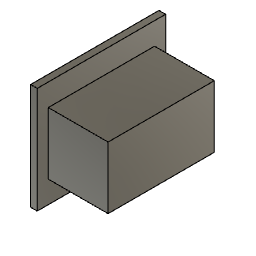
Assembly v11 (Autodesk Fusion 360 archive; units mm, degrees)
design "Power"
Autodesk Fusion 360 part; units mm, degrees
sketch "Sketch1" plane through (0, 0, 0) normal (1, 0, 0) x (0, 1, 0)
  line L0 (0, 0) -> (48, 0)
  line L1 (48, 0) -> (48, 28)
  line L2 (48, 28) -> (0, 28)
  line L3 (0, 28) -> (0, 0)
  dimension "d1" = 48
  dimension "d2" = 28
  constraint horizontal L0
  constraint vertical L1
  constraint horizontal L2
  constraint vertical L3
  constraint coincident L0.start L3.end
  measures "d1" distance of L0.start L0.end
  measures "d2" distance of L0.start L2.end
extrude "Extrude1" add sketch "Sketch1" along normal blind 27
sketch "Sketch2" plane through (0, 0, 0) normal (-1, 0, 0) x (0, -1, 0)
  line L0 (0, 0) -> (0, 28)
  line L1 (0, 28) -> (-48, 28)
  line L2 (-48, 28) -> (-48, 0)
  line L3 (-48, 0) -> (0, 0)
  line L4 (-48, 28) -> (0, 0) construction
  line L5 (0, 28) -> (-48, 0) construction
  line L6 (5, -10) -> (-53, -10)
  line L7 (-53, -10) -> (-53, 38)
  line L8 (-53, 38) -> (5, 38)
  line L9 (5, 38) -> (5, -10)
  line L10 (5, -10) -> (-53, 38) construction
  line L11 (-53, -10) -> (5, 38) construction
  point P0 (-24, 14)
  dimension "d5" = 58
  dimension "d6" = 48
  constraint coincident L1.end L2.start
  constraint coincident L0.start L3.end
  constraint coincident L0.end L1.start
  constraint coincident L2.end L3.start
  constraint horizontal L6
  constraint perpendicular L6 L7
  constraint parallel L6 L8
  constraint parallel L7 L9
  constraint coincident L10 P0
  constraint coincident L11 P0
  constraint midpoint L5 P0
  measures "d5" distance of L7.end L8.end
  measures "d6" distance of L6.end L7.end
extrude "Extrude2" add sketch "Sketch2" along normal blind 3 contours L0 L1 L2 L3 | L6 L7 L8 L9

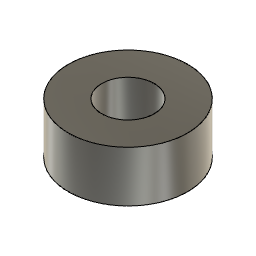
design "Transfo"
Autodesk Fusion 360 part; units mm, degrees
sketch "Sketch1" plane through (0, 0, 0) normal (0, 0, 1) x (1, 0, 0)
  circle A0 centre (0, 0) radius 37.5
  circle A1 centre (0, 0) radius 16.5
  dimension "d1" = 75
  dimension "d2" = 33
  constraint coincident A0.centre A1.centre
  constraint concentric A0 A1
  measures "d1" diameter of A0
  measures "d2" diameter of A1
extrude "Extrude1" add sketch "Sketch1" along normal blind 32

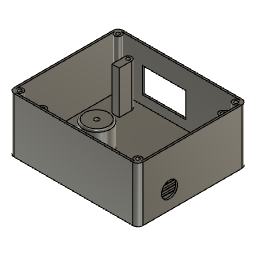
design "Case"
Autodesk Fusion 360 part; units mm, degrees
sketch "CASE" plane through (0, 0, 0) normal (0, 0, 1) x (1, 0, 0)
  line L0 (0, 0) -> (125, 0)
  line L1 (125, 0) -> (125, 104)
  line L2 (125, 104) -> (0, 104)
  line L3 (0, 104) -> (0, 0)
  line L4 (0, 104) -> (125, 0) construction
  line L5 (125, 104) -> (0, 0) construction
  line L6 (112.0817, 93.252) -> (147.6564, 122.8501) construction
  circle A0 centre (128.0749, 106.5583) radius 2
  line L7 (62.5, 54.9936) -> (62.5, 47.4797) construction
  line L8 (60.7161, 52) -> (65.2538, 52) construction
  line L9 (12.9183, 93.252) -> (-22.6564, 122.8501) construction
  circle A1 centre (-3.0749, 106.5583) radius 2
  circle A2 centre (-3.0749, -2.5583) radius 2
  line L10 (12.9183, 10.748) -> (-22.6564, -18.8501) construction
  line L11 (112.0817, 10.748) -> (147.6564, -18.8501) construction
  circle A3 centre (128.0749, -2.5583) radius 2
  line L12 (-3.0749, 110.5583) -> (128.0749, 110.5583)
  line L13 (-3.0749, -6.5583) -> (128.0749, -6.5583)
  line L14 (-7.0749, -2.5583) -> (-7.0749, -7.9197) construction
  line L15 (132.0749, -2.5583) -> (132.0749, -5.8863) construction
  line L16 (134.0749, -2.8083) -> (134.0749, 106.8083)
  line L17 (-3.3249, 112.5583) -> (128.3249, 112.5583)
  line L18 (-9.0749, -2.8083) -> (-9.0749, 106.8083)
  line L19 (-3.3249, -8.5583) -> (128.3249, -8.5583)
  line L20 (-7.0749, -2.5583) -> (-7.0749, 106.5583)
  line L21 (132.0749, -2.5583) -> (132.0749, 106.5583)
  arc A4 (-3.3249, 112.5583) -> (-9.0749, 106.8083) centre (-3.3249, 106.8083) ccw
  arc A5 (-9.0749, -2.8083) -> (-3.3249, -8.5583) centre (-3.3249, -2.8083) ccw
  arc A6 (128.3249, -8.5583) -> (134.0749, -2.8083) centre (128.3249, -2.8083) ccw
  arc A7 (134.0749, 106.8083) -> (128.3249, 112.5583) centre (128.3249, 106.8083) ccw
  arc A8 (128.0749, 110.5583) -> (132.0749, 106.5583) centre (128.0749, 106.5583) ccw
  arc A9 (-7.0749, 106.5583) -> (-3.0749, 110.5583) centre (-3.0749, 106.5583) ccw
  arc A10 (-3.0749, -6.5583) -> (-7.0749, -2.5583) centre (-3.0749, -2.5583) ccw
  arc A11 (132.0749, -2.5583) -> (128.0749, -6.5583) centre (128.0749, -2.5583) ccw
  dimension "d1" = 125
  dimension "d2" = 104
  dimension "d3" = 8
  dimension "d4" = 4
  dimension "d6" = 5.75
  dimension "d7" = 5.75
  dimension "d8" = 5.75
  dimension "d9" = 5.75
  constraint horizontal L0
  constraint vertical L1
  constraint horizontal L2
  constraint vertical L3
  constraint coincident L0.start L3.end
  constraint coincident L5 L6.start
  constraint parallel L5 L6
  constraint coincident L6 A0.centre
  constraint concentric A0 A8
  constraint coincident L1.end A8
  constraint vertical L7
  constraint perpendicular L7 L8
  constraint symmetric L6.start L7 L9.start
  constraint symmetric L6.end L7 L9.end
  constraint symmetric L7 A8 A9
  constraint symmetric A0 L7 A1
  constraint symmetric L6.start L8 L11.start
  constraint symmetric L6.end L8 L11.end
  constraint symmetric L8 A8 A11
  constraint symmetric A0 L8 A3
  constraint symmetric L8 A9 A10
  constraint symmetric L8 L9.start L10.start
  constraint symmetric L8 L9.end L10.end
  constraint symmetric L8 A1 A2
  constraint horizontal L12
  constraint tangent L12 A8
  constraint horizontal L13
  constraint tangent L13 A11
  constraint coincident L0.start A10
  constraint tangent L14 A10
  constraint perpendicular L13 L14
  constraint perpendicular L12 L20
  constraint tangent L15 A11
  constraint perpendicular L13 L15
  constraint parallel L12 L17
  constraint parallel L18 L20
  constraint parallel L13 L19
  constraint coincident L11 L15.end
  constraint tangent L17 A4
  constraint tangent L18 A4
  constraint tangent L18 A5
  constraint tangent L19 A5
  constraint tangent L16 A6
  constraint tangent L19 A6
  constraint tangent L17 A7
  constraint tangent L16 A7
  measures "d1" distance of L0.start L0.end
  measures "d2" distance of L0.start L2.end
  measures "d3" diameter of A8
  measures "d4" diameter of A0
  measures "d6" radius of A4
  measures "d7" radius of A5
  measures "d8" radius of A6
  measures "d9" radius of A7
extrude "Extrude1" add sketch "CASE" along normal blind 61
extrude "Extrude2" add sketch "CASE" along normal blind 2 contours L0 L1 L2 L3 | L3 L20 A9 A10 | L0 L13 A10 A11 | L1 L21 A8 A11 | L2 L12 A8 A9
extrude "Extrude3" add sketch "CASE" along normal up to surface (55 mm away) contours A0 | A1 | A2 | A3
sketch "PCB MOUNT" plane through (0, 0, 2) normal (0, 0, 1) x (-1, 0, 0)
  line L0 (3.0749, 6.5583) -> (-128.0749, 6.5583)
  arc A0 (-132.0749, 2.5583) -> (-128.0749, 6.5583) centre (-128.0749, 2.5583) ccw
  line L1 (-132.0749, 2.5583) -> (-132.0749, -106.5583)
  arc A1 (-128.0749, -110.5583) -> (-132.0749, -106.5583) centre (-128.0749, -106.5583) ccw
  line L2 (-128.0749, -110.5583) -> (3.0749, -110.5583)
  arc A2 (7.0749, -106.5583) -> (3.0749, -110.5583) centre (3.0749, -106.5583) ccw
  line L3 (7.0749, -106.5583) -> (7.0749, 2.5583)
  arc A3 (3.0749, 6.5583) -> (7.0749, 2.5583) centre (3.0749, 2.5583) ccw
  line L4 (0, 0) -> (-125, 0) construction
  line L5 (-125, 0) -> (-125, -104) construction
  line L6 (-125, -104) -> (0, -104) construction
  line L7 (0, -104) -> (0, 0) construction
  line L8 (0, -104) -> (-125, 0) construction
  line L9 (-125, -104) -> (0, 0) construction
  circle A4 centre (-15.1125, -99.625) radius 2
  circle A5 centre (-119.8875, -99.625) radius 2
  circle A6 centre (-119.8875, -99.625) radius 4
  circle A7 centre (-15.1125, -4.375) radius 4
  circle A8 centre (-15.1125, -4.375) radius 2
  circle A9 centre (-119.8875, -4.375) radius 2
  circle A10 centre (-119.8875, -4.375) radius 4
  line L10 (-62.5, -55.0458) -> (-62.5, -45.3587) construction
  line L11 (-59.1792, -52) -> (-68.8663, -52) construction
  line L12 (-19.1125, -99.625) -> (-19.1125, -85.625)
  line L13 (-19.1125, -85.625) -> (-11.1125, -85.625)
  line L14 (-11.1125, -85.625) -> (-11.1125, -99.625)
  arc A11 (-19.1125, -99.625) -> (-11.1125, -99.625) centre (-15.1125, -99.625) ccw
  dimension "d16" = 125
  dimension "d17" = 104
  dimension "d18" = 8
  dimension "d19" = 4
  dimension "d20" = 8
  dimension "d21" = 4
  dimension "d22" = 8
  dimension "d23" = 4
  dimension "d24" = 8
  dimension "d25" = 4
  dimension "d26" = 104.775
  dimension "d27" = 95.25
  dimension "d28" = 47.3875
  dimension "d29" = 47.625
  dimension "d48" = 14
  constraint horizontal L4
  constraint vertical L5
  constraint horizontal L6
  constraint vertical L7
  constraint coincident L4.start L7.end
  constraint concentric A4 A11
  constraint concentric A5 A6
  constraint concentric A7 A8
  constraint concentric A9 A10
  constraint vertical A5.centre A9.centre
  constraint vertical A4.centre A7.centre
  constraint horizontal A7.centre A9.centre
  constraint horizontal A4.centre A5.centre
  constraint perpendicular L6 L10
  constraint parallel L2 L11
  constraint vertical L12
  constraint horizontal L13
  constraint vertical L14
  constraint tangent L12 A11
  measures "d16" distance of L4.start L4.end
  measures "d17" distance of L4.start L6.end
  measures "d18" diameter of A11
  measures "d19" diameter of A4
  measures "d20" diameter of A6
  measures "d21" diameter of A5
  measures "d22" diameter of A7
  measures "d23" diameter of A8
  measures "d24" diameter of A10
  measures "d25" diameter of A9
  measures "d26" distance of A4.centre A5.centre
  measures "d27" distance of A4.centre A7.centre
  measures "d28" distance of A4.centre L10
  measures "d29" distance of A4.centre L11
  measures "d48" distance of L14.end L13.end
extrude "Extrude4" add sketch "PCB MOUNT" along normal blind 47.5 contours A6 | A7 | A10 | L12 L13 L14 A11
extrude "Extrude5" add sketch "PCB MOUNT" along normal up to surface (41.5 mm away) contours A4 | A5 | A8 | A9
sketch "TRANS" plane through (0, 0, 2) normal (0, 0, 1) x (-1, 0, 0)
  circle A0 centre (-119.8875, -99.625) radius 4
  line L0 (3.0749, 6.5583) -> (-128.0749, 6.5583)
  arc A1 (-132.0749, 2.5583) -> (-128.0749, 6.5583) centre (-128.0749, 2.5583) ccw
  line L1 (-132.0749, 2.5583) -> (-132.0749, -106.5583)
  arc A2 (-128.0749, -110.5583) -> (-132.0749, -106.5583) centre (-128.0749, -106.5583) ccw
  line L2 (-128.0749, -110.5583) -> (3.0749, -110.5583)
  arc A3 (7.0749, -106.5583) -> (3.0749, -110.5583) centre (3.0749, -106.5583) ccw
  line L3 (7.0749, -106.5583) -> (7.0749, 2.5583)
  arc A4 (3.0749, 6.5583) -> (7.0749, 2.5583) centre (3.0749, 2.5583) ccw
  circle A5 centre (-15.1125, -4.375) radius 4
  circle A6 centre (-119.8875, -4.375) radius 4
  circle A7 centre (-36.3235, -43.5484) radius 37.5 construction
  circle A8 centre (-36.3235, -43.5484) radius 15
  line L4 (-19.1125, -85.625) -> (-11.1125, -85.625)
  line L5 (-11.1125, -85.625) -> (-11.1125, -99.625)
  arc A9 (-19.1125, -99.625) -> (-11.1125, -99.625) centre (-15.1125, -99.625) ccw
  line L6 (-19.1125, -99.625) -> (-19.1125, -85.625)
  dimension "d36" = 75
  dimension "d37" = 30
  constraint concentric A7 A8
  measures "d36" diameter of A7
  measures "d37" diameter of A8
extrude "Extrude6" add sketch "TRANS" along normal blind 28 contours A8
fillet "Fillet1" radius 2 1 edges at (50.3084, 48.9727, 30)
sketch "TRANSMOUNT" plane through (0, 0, 30) normal (0, 0, 1) x (-1, 0, 0)
  circle A0 centre (-36.3235, -43.5484) radius 13
  point P0 (-36.3235, -43.5484)
  constraint coincident P0 A0.centre
hole "Hole1" at (36.3235, 43.5484, 30) direction (0, 0, -1) diameter 5 end through all
sketch "TRANSNUT" plane through (0, 0, 0) normal (0, 0, -1) x (1, 0, 0)
  circle A0 centre (36.3235, -43.5484) radius 2.5
  arc A1 (-3.3249, 8.5583) -> (-9.0749, 2.8083) centre (-3.3249, 2.8083) ccw
  line L0 (-9.0749, 2.8083) -> (-9.0749, -106.8083)
  arc A2 (-9.0749, -106.8083) -> (-3.3249, -112.5583) centre (-3.3249, -106.8083) ccw
  line L1 (-3.3249, -112.5583) -> (128.3249, -112.5583)
  arc A3 (128.3249, -112.5583) -> (134.0749, -106.8083) centre (128.3249, -106.8083) ccw
  line L2 (134.0749, -106.8083) -> (134.0749, 2.8083)
  arc A4 (134.0749, 2.8083) -> (128.3249, 8.5583) centre (128.3249, 2.8083) ccw
  line L3 (128.3249, 8.5583) -> (-3.3249, 8.5583)
  line L4 (40.5611, -41.1898) -> (36.3997, -38.6993)
  line L5 (36.3997, -38.6993) -> (32.1621, -41.0579)
  line L6 (32.1621, -41.0579) -> (32.086, -45.907)
  line L7 (32.086, -45.907) -> (36.2473, -48.3976)
  line L8 (36.2473, -48.3976) -> (40.4849, -46.039)
  line L9 (40.4849, -46.039) -> (40.5611, -41.1898)
  point P0 (36.3235, -43.5484)
  dimension "d45" = 4.2
  constraint coincident P0 A0.centre
  measures "d45" distance of P0 L9
extrude "Extrude7" cut sketch "TRANSNUT" against normal blind 4.5 contours L4 L5 L6 L7 L8 L9
sketch "POWER" plane through (0, 112.5583, 0) normal (0, 1, 0) x (-1, 0, 0)
  line L0 (-128.3249, 0) -> (3.3249, 0)
  line L1 (3.3249, 0) -> (3.3249, 61)
  line L2 (3.3249, 61) -> (-128.3249, 61)
  line L3 (-128.3249, 61) -> (-128.3249, 0)
  line L4 (-67.9251, 40) -> (-19.9251, 40)
  line L5 (-19.9251, 40) -> (-19.9251, 12)
  line L6 (-19.9251, 12) -> (-67.9251, 12)
  line L7 (-67.9251, 12) -> (-67.9251, 40)
  line L8 (-67.9251, 40) -> (-19.9251, 12) construction
  line L9 (-19.9251, 40) -> (-67.9251, 12) construction
  line L10 (9.0749, 0) -> (9.0749, 61) construction
  point P0 (-43.9251, 26)
  dimension "d55" = 48
  dimension "d56" = 28
  dimension "d57" = 35
  dimension "d58" = 53
  constraint horizontal L4
  constraint vertical L5
  constraint horizontal L6
  constraint vertical L7
  constraint midpoint L9 P0
  measures "d55" distance of L4.start L4.end
  measures "d56" distance of L4.start L6.end
  measures "d57" distance of L2 P0
  measures "d58" distance of P0 L10
extrude "Extrude9" cut sketch "POWER" against normal up to surface (2 mm away) contours L4 L5 L6 L7
sketch "VENTS" plane through (0, 0, 2) normal (0, 0, 1) x (-1, 0, 0)
  circle A0 centre (-36.3235, -43.5484) radius 15
  line L0 (-19.1125, -85.625) -> (-11.1125, -85.625)
  line L1 (-11.1125, -85.625) -> (-11.1125, -99.625)
  arc A1 (-19.1125, -99.625) -> (-11.1125, -99.625) centre (-15.1125, -99.625) ccw
  line L2 (-19.1125, -99.625) -> (-19.1125, -85.625)
  circle A2 centre (-119.8875, -99.625) radius 4
  line L3 (3.0749, 6.5583) -> (-128.0749, 6.5583)
  arc A3 (-132.0749, 2.5583) -> (-128.0749, 6.5583) centre (-128.0749, 2.5583) ccw
  line L4 (-132.0749, 2.5583) -> (-132.0749, -106.5583)
  arc A4 (-128.0749, -110.5583) -> (-132.0749, -106.5583) centre (-128.0749, -106.5583) ccw
  line L5 (-128.0749, -110.5583) -> (3.0749, -110.5583)
  arc A5 (7.0749, -106.5583) -> (3.0749, -110.5583) centre (3.0749, -106.5583) ccw
  line L6 (7.0749, -106.5583) -> (7.0749, 2.5583)
  arc A6 (3.0749, 6.5583) -> (7.0749, 2.5583) centre (3.0749, 2.5583) ccw
  circle A7 centre (-15.1125, -4.375) radius 4
  circle A8 centre (-119.8875, -4.375) radius 4
  line L7 (-62.0749, -86.9998) -> (-122.0749, -86.9998) construction
  line L8 (-122.0749, -86.9998) -> (-122.0749, -16.9998) construction
  line L9 (-122.0749, -16.9998) -> (-62.0749, -16.9998) construction
  line L10 (-62.0749, -86.9998) -> (-122.0749, -16.9998) construction
  line L11 (-122.0749, -86.9998) -> (-62.0749, -16.9998) construction
  arc A9 (-78.3249, -86.9998) -> (-77.0749, -85.7498) centre (-78.3249, -85.7498) ccw
  line L12 (-79.5749, -85.7498) -> (-79.5749, -18.2498)
  line L13 (-77.0749, -16.9998) -> (-77.0749, -86.9998) construction
  line L14 (-77.0749, -18.2498) -> (-77.0749, -85.7498)
  arc A10 (-79.5749, -85.7498) -> (-78.3249, -86.9998) centre (-78.3249, -85.7498) ccw
  arc A11 (-77.0749, -18.2498) -> (-78.3249, -16.9998) centre (-78.3249, -18.2498) ccw
  arc A12 (-78.3249, -16.9998) -> (-79.5749, -18.2498) centre (-78.3249, -18.2498) ccw
  line L15 (-89.5749, -85.7498) -> (-89.5749, -18.2498)
  arc A13 (-87.0749, -18.2498) -> (-88.3249, -16.9998) centre (-88.3249, -18.2498) ccw
  arc A14 (-82.0749, -18.2498) -> (-83.3249, -16.9998) centre (-83.3249, -18.2498) ccw
  arc A15 (-93.3249, -16.9998) -> (-94.5749, -18.2498) centre (-93.3249, -18.2498) ccw
  line L16 (-94.5749, -85.7498) -> (-94.5749, -18.2498)
  line L17 (-78.3249, -16.9998) -> (-78.3249, -16.9998)
  arc A16 (-83.3249, -86.9998) -> (-82.0749, -85.7498) centre (-83.3249, -85.7498) ccw
  arc A17 (-98.3249, -16.9998) -> (-99.5749, -18.2498) centre (-98.3249, -18.2498) ccw
  line L18 (-99.5749, -85.7498) -> (-99.5749, -18.2498)
  arc A18 (-89.5749, -85.7498) -> (-88.3249, -86.9998) centre (-88.3249, -85.7498) ccw
  arc A19 (-84.5749, -85.7498) -> (-83.3249, -86.9998) centre (-83.3249, -85.7498) ccw
  line L19 (-92.0749, -16.9998) -> (-92.0749, -86.9998) construction
  arc A20 (-88.3249, -86.9998) -> (-87.0749, -85.7498) centre (-88.3249, -85.7498) ccw
  line L20 (-97.0749, -16.9998) -> (-97.0749, -86.9998) construction
  arc A21 (-88.3249, -16.9998) -> (-89.5749, -18.2498) centre (-88.3249, -18.2498) ccw
  arc A22 (-92.0749, -18.2498) -> (-93.3249, -16.9998) centre (-93.3249, -18.2498) ccw
  line L21 (-97.0749, -18.2498) -> (-97.0749, -85.7498)
  line L22 (-92.0749, -18.2498) -> (-92.0749, -85.7498)
  line L23 (-84.5749, -85.7498) -> (-84.5749, -18.2498)
  arc A23 (-97.0749, -18.2498) -> (-98.3249, -16.9998) centre (-98.3249, -18.2498) ccw
  arc A24 (-83.3249, -16.9998) -> (-84.5749, -18.2498) centre (-83.3249, -18.2498) ccw
  arc A25 (-93.3249, -86.9998) -> (-92.0749, -85.7498) centre (-93.3249, -85.7498) ccw
  line L24 (-87.0749, -16.9998) -> (-87.0749, -86.9998) construction
  line L25 (-82.0749, -16.9998) -> (-82.0749, -86.9998) construction
  arc A26 (-98.3249, -86.9998) -> (-97.0749, -85.7498) centre (-98.3249, -85.7498) ccw
  arc A27 (-99.5749, -85.7498) -> (-98.3249, -86.9998) centre (-98.3249, -85.7498) ccw
  line L26 (-78.3249, -86.9998) -> (-78.3249, -86.9998)
  arc A28 (-94.5749, -85.7498) -> (-93.3249, -86.9998) centre (-93.3249, -85.7498) ccw
  line L27 (-82.0749, -18.2498) -> (-82.0749, -85.7498)
  line L28 (-87.0749, -18.2498) -> (-87.0749, -85.7498)
  line L29 (-109.5749, -85.7498) -> (-109.5749, -18.2498)
  arc A29 (-107.0749, -18.2498) -> (-108.3249, -16.9998) centre (-108.3249, -18.2498) ccw
  arc A30 (-102.0749, -18.2498) -> (-103.3249, -16.9998) centre (-103.3249, -18.2498) ccw
  arc A31 (-113.3249, -16.9998) -> (-114.5749, -18.2498) centre (-113.3249, -18.2498) ccw
  line L30 (-114.5749, -85.7498) -> (-114.5749, -18.2498)
  line L31 (-78.3249, -16.9998) -> (-78.3249, -16.9998)
  arc A32 (-103.3249, -86.9998) -> (-102.0749, -85.7498) centre (-103.3249, -85.7498) ccw
  arc A33 (-118.3249, -16.9998) -> (-119.5749, -18.2498) centre (-118.3249, -18.2498) ccw
  line L32 (-119.5749, -85.7498) -> (-119.5749, -18.2498)
  arc A34 (-109.5749, -85.7498) -> (-108.3249, -86.9998) centre (-108.3249, -85.7498) ccw
  arc A35 (-104.5749, -85.7498) -> (-103.3249, -86.9998) centre (-103.3249, -85.7498) ccw
  line L33 (-112.0749, -16.9998) -> (-112.0749, -86.9998) construction
  arc A36 (-108.3249, -86.9998) -> (-107.0749, -85.7498) centre (-108.3249, -85.7498) ccw
  line L34 (-117.0749, -16.9998) -> (-117.0749, -86.9998) construction
  arc A37 (-108.3249, -16.9998) -> (-109.5749, -18.2498) centre (-108.3249, -18.2498) ccw
  arc A38 (-112.0749, -18.2498) -> (-113.3249, -16.9998) centre (-113.3249, -18.2498) ccw
  line L35 (-117.0749, -18.2498) -> (-117.0749, -85.7498)
  line L36 (-112.0749, -18.2498) -> (-112.0749, -85.7498)
  line L37 (-104.5749, -85.7498) -> (-104.5749, -18.2498)
  arc A39 (-117.0749, -18.2498) -> (-118.3249, -16.9998) centre (-118.3249, -18.2498) ccw
  arc A40 (-103.3249, -16.9998) -> (-104.5749, -18.2498) centre (-103.3249, -18.2498) ccw
  arc A41 (-113.3249, -86.9998) -> (-112.0749, -85.7498) centre (-113.3249, -85.7498) ccw
  line L38 (-107.0749, -16.9998) -> (-107.0749, -86.9998) construction
  line L39 (-102.0749, -16.9998) -> (-102.0749, -86.9998) construction
  arc A42 (-118.3249, -86.9998) -> (-117.0749, -85.7498) centre (-118.3249, -85.7498) ccw
  arc A43 (-119.5749, -85.7498) -> (-118.3249, -86.9998) centre (-118.3249, -85.7498) ccw
  line L40 (-78.3249, -86.9998) -> (-78.3249, -86.9998)
  arc A44 (-114.5749, -85.7498) -> (-113.3249, -86.9998) centre (-113.3249, -85.7498) ccw
  line L41 (-102.0749, -18.2498) -> (-102.0749, -85.7498)
  line L42 (-107.0749, -18.2498) -> (-107.0749, -85.7498)
  point P0 (-92.0749, -51.9998)
  point P1 (-79.5749, -86.9998)
  point P2 (-77.0749, -16.9998)
  point P3 (-99.5749, -86.9998)
  point P4 (-97.0749, -16.9998)
  point P5 (-94.5749, -86.9998)
  point P6 (-92.0749, -16.9998)
  point P7 (-84.5749, -86.9998)
  point P8 (-82.0749, -16.9998)
  point P9 (-89.5749, -86.9998)
  point P10 (-87.0749, -16.9998)
  point P11 (-119.5749, -86.9998)
  point P12 (-117.0749, -16.9998)
  point P13 (-114.5749, -86.9998)
  point P14 (-112.0749, -16.9998)
  point P15 (-104.5749, -86.9998)
  point P16 (-102.0749, -16.9998)
  point P17 (-109.5749, -86.9998)
  point P18 (-107.0749, -16.9998)
  dimension "d193" = 60
  dimension "d194" = 70
  dimension "d195" = 58.5585
  dimension "d196" = 40
  dimension "d249" = 70
  dimension "d250" = 2.5
  dimension "d251" = 70
  dimension "d252" = 1.25
  dimension "d254" = 70
  dimension "d255" = 2.5
  dimension "d256" = 70
  dimension "d257" = 1.25
  dimension "d258" = 70
  dimension "d259" = 2.5
  dimension "d260" = 70
  dimension "d261" = 1.25
  dimension "d262" = 5
  dimension "d263" = 70
  dimension "d264" = 2.5
  dimension "d265" = 70
  dimension "d266" = 1.25
  dimension "d267" = 70
  dimension "d268" = 2.5
  dimension "d269" = 70
  dimension "d270" = 1.25
  dimension "d271" = 5
  dimension "d272" = 70
  dimension "d273" = 2.5
  dimension "d274" = 70
  dimension "d275" = 1.25
  dimension "d276" = 70
  dimension "d277" = 2.5
  dimension "d278" = 70
  dimension "d279" = 1.25
  dimension "d280" = 5
  dimension "d281" = 70
  dimension "d282" = 2.5
  dimension "d283" = 70
  dimension "d284" = 1.25
  dimension "d285" = 70
  dimension "d286" = 2.5
  dimension "d287" = 70
  dimension "d288" = 1.25
  dimension "d289" = 5
  constraint horizontal L7
  constraint vertical L8
  constraint horizontal L9
  constraint midpoint L10 P0
  constraint vertical L13
  constraint vertical L12
  constraint vertical L14
  constraint coincident L13.end L14
  constraint tangent A9 L14
  constraint coincident P1 L12
  constraint tangent L12 A10
  constraint equal A9 A10
  constraint tangent L12 A12
  constraint equal A9 A12
  constraint coincident P2 L14
  constraint tangent L14 A11
  constraint equal A9 A11
  constraint vertical L25
  constraint vertical L23
  constraint vertical L27
  constraint coincident L25.end L27
  constraint tangent A16 L27
  constraint coincident P7 L23
  constraint tangent A19 L23
  constraint equal A16 A19
  constraint tangent L23 A24
  constraint equal A16 A24
  constraint coincident P8 L27
  constraint tangent A14 L27
  constraint equal A14 A16
  constraint vertical L24
  constraint vertical L15
  constraint vertical L28
  constraint coincident L24.end L28
  constraint tangent A20 L28
  constraint coincident P9 L15
  constraint tangent L15 A18
  constraint equal A18 A20
  constraint tangent L15 A21
  constraint equal A20 A21
  constraint coincident P10 L28
  constraint tangent A13 L28
  constraint equal A13 A20
  constraint vertical L19
  constraint vertical L16
  constraint vertical L22
  constraint coincident L19.end L22
  constraint tangent L22 A25
  constraint coincident P5 L16
  constraint tangent L16 A28
  constraint equal A25 A28
  constraint tangent A15 L16
  constraint equal A15 A25
  constraint coincident P6 L22
  constraint tangent A22 L22
  constraint equal A22 A25
  constraint vertical L20
  constraint vertical L18
  constraint vertical L21
  constraint coincident L20.end L21
  constraint tangent L21 A26
  constraint coincident P3 L18
  constraint coincident P3 L26
  constraint tangent L18 A27
  constraint equal A26 A27
  constraint tangent A17 L18
  constraint equal A17 A26
  constraint coincident P4 L21
  constraint coincident P4 L17
  constraint tangent L21 A23
  constraint equal A23 A26
  constraint vertical L39
  constraint vertical L37
  constraint vertical L41
  constraint coincident L39.end L41
  constraint tangent A32 L41
  constraint coincident P15 L37
  constraint tangent A35 L37
  constraint equal A32 A35
  constraint tangent L37 A40
  constraint equal A32 A40
  constraint coincident P16 L41
  constraint tangent A30 L41
  constraint equal A30 A32
  constraint vertical L38
  constraint vertical L29
  constraint vertical L42
  constraint coincident L38.end L42
  constraint tangent A36 L42
  constraint coincident P17 L29
  constraint tangent L29 A34
  constraint equal A34 A36
  constraint tangent L29 A37
  constraint equal A36 A37
  constraint coincident P18 L42
  constraint tangent A29 L42
  constraint equal A29 A36
  constraint vertical L33
  constraint vertical L30
  constraint vertical L36
  constraint coincident L33.end L36
  constraint tangent L36 A41
  constraint coincident P13 L30
  constraint tangent L30 A44
  constraint equal A41 A44
  constraint tangent A31 L30
  constraint equal A31 A41
  constraint coincident P14 L36
  constraint tangent A38 L36
  constraint equal A38 A41
  constraint vertical L34
  constraint vertical L32
  constraint vertical L35
  constraint coincident L34.end L35
  constraint tangent L35 A42
  constraint coincident P11 L32
  constraint coincident P11 L40
  constraint tangent L32 A43
  constraint equal A42 A43
  constraint tangent A33 L32
  constraint equal A33 A42
  constraint coincident P12 L35
  constraint coincident P12 L31
  constraint tangent L35 A39
  constraint equal A39 A42
  measures "d193" distance of L7.start L7.end
  measures "d194" distance of L7.start L9.end
  measures "d195" distance of L5 P0
  measures "d196" distance of L4 P0
  measures "d249" distance of L13.end P2
  measures "d250" distance of L13.end P1
  measures "d251" distance of L13.end P2
  measures "d252" radius of A9
  measures "d254" distance of P8 L25.end
  measures "d255" distance of P7 L25.end
  measures "d256" distance of P8 L25.end
  measures "d257" radius of A16
  measures "d258" distance of L24.end P10
  measures "d259" distance of L24.end P9
  measures "d260" distance of L24.end P10
  measures "d261" radius of A20
  measures "d262" distance of A18.centre A16.centre
  measures "d263" distance of L19.end P6
  measures "d264" distance of P5 L19.end
  measures "d265" distance of P6 L19.end
  measures "d266" radius of A25
  measures "d267" distance of P4 L20.end
  measures "d268" distance of P3 L20.end
  measures "d269" distance of P4 L20.end
  measures "d270" radius of A26
  measures "d271" distance of A25.centre A26.centre
  measures "d272" distance of P16 L39.end
  measures "d273" distance of P15 L39.end
  measures "d274" distance of P16 L39.end
  measures "d275" radius of A32
  measures "d276" distance of L38.end P18
  measures "d277" distance of L38.end P17
  measures "d278" distance of L38.end P18
  measures "d279" radius of A36
  measures "d280" distance of A34.centre A32.centre
  measures "d281" distance of L33.end P14
  measures "d282" distance of P13 L33.end
  measures "d283" distance of P14 L33.end
  measures "d284" radius of A41
  measures "d285" distance of P12 L34.end
  measures "d286" distance of P11 L34.end
  measures "d287" distance of P12 L34.end
  measures "d288" radius of A42
  measures "d289" distance of A41.centre A42.centre
extrude "Extrude10" cut sketch "VENTS" against normal up to surface (2 mm away) contours A9 L12 L14 A10 A11 A12 | L15 A13 A18 A20 A21 L28 | A14 A16 A19 L23 A24 L27 | A15 L16 A22 L22 A25 A28 | A17 L18 L21 A23 A26 A27 | L29 A29 A34 A36 A37 L42 | A30 A32 A35 L37 A40 L41 | A31 L30 A38 L36 A41 A44 | A33 L32 L35 A39 A42 A43
sketch "CONNECTOR" plane through (134.0749, 0, 0) normal (1, 0, 0) x (0, 1, 0)
  line L0 (-2.8083, 0) -> (106.8083, 0)
  line L1 (106.8083, 0) -> (106.8083, 61)
  line L2 (106.8083, 61) -> (-2.8083, 61)
  line L3 (-2.8083, 61) -> (-2.8083, 0)
  circle A0 centre (26.4417, 20) radius 9
  line L4 (-8.5583, 0) -> (-8.5583, 61)
  dimension "d290" = 18
  dimension "d291" = 35
  dimension "d292" = 20
  measures "d290" diameter of A0
  measures "d291" distance of A0.centre L4
  measures "d292" distance of L0 A0.centre
extrude "Extrude11" cut sketch "CONNECTOR" against normal up to surface (2 mm away) contours A0
sketch "STRENGHTEN" plane through (0, 0, 2) normal (0, 0, 1) x (-1, 0, 0)
  line L0 (-107.0749, -18.2498) -> (-107.0749, -85.7498)
  arc A0 (-109.5749, -85.7498) -> (-107.0749, -85.7498) centre (-108.3249, -85.7498) ccw
  line L1 (-109.5749, -85.7498) -> (-109.5749, -18.2498)
  arc A1 (-107.0749, -18.2498) -> (-109.5749, -18.2498) centre (-108.3249, -18.2498) ccw
  line L2 (-87.0749, -18.2498) -> (-87.0749, -85.7498)
  arc A2 (-89.5749, -85.7498) -> (-87.0749, -85.7498) centre (-88.3249, -85.7498) ccw
  line L3 (-89.5749, -85.7498) -> (-89.5749, -18.2498)
  arc A3 (-87.0749, -18.2498) -> (-89.5749, -18.2498) centre (-88.3249, -18.2498) ccw
  line L4 (-82.0749, -18.2498) -> (-82.0749, -85.7498)
  arc A4 (-84.5749, -85.7498) -> (-82.0749, -85.7498) centre (-83.3249, -85.7498) ccw
  line L5 (-84.5749, -85.7498) -> (-84.5749, -18.2498)
  arc A5 (-82.0749, -18.2498) -> (-84.5749, -18.2498) centre (-83.3249, -18.2498) ccw
  line L6 (-102.0749, -18.2498) -> (-102.0749, -85.7498)
  arc A6 (-104.5749, -85.7498) -> (-102.0749, -85.7498) centre (-103.3249, -85.7498) ccw
  line L7 (-104.5749, -85.7498) -> (-104.5749, -18.2498)
  arc A7 (-102.0749, -18.2498) -> (-104.5749, -18.2498) centre (-103.3249, -18.2498) ccw
  line L8 (-112.0749, -18.2498) -> (-112.0749, -85.7498)
  arc A8 (-114.5749, -85.7498) -> (-112.0749, -85.7498) centre (-113.3249, -85.7498) ccw
  line L9 (-114.5749, -85.7498) -> (-114.5749, -18.2498)
  arc A9 (-112.0749, -18.2498) -> (-114.5749, -18.2498) centre (-113.3249, -18.2498) ccw
  line L10 (-92.0749, -18.2498) -> (-92.0749, -85.7498)
  arc A10 (-94.5749, -85.7498) -> (-92.0749, -85.7498) centre (-93.3249, -85.7498) ccw
  line L11 (-94.5749, -85.7498) -> (-94.5749, -18.2498)
  arc A11 (-92.0749, -18.2498) -> (-94.5749, -18.2498) centre (-93.3249, -18.2498) ccw
  line L12 (-77.0749, -18.2498) -> (-77.0749, -85.7498)
  arc A12 (-79.5749, -85.7498) -> (-77.0749, -85.7498) centre (-78.3249, -85.7498) ccw
  line L13 (-79.5749, -85.7498) -> (-79.5749, -18.2498)
  arc A13 (-77.0749, -18.2498) -> (-79.5749, -18.2498) centre (-78.3249, -18.2498) ccw
  line L14 (-97.0749, -18.2498) -> (-97.0749, -85.7498)
  arc A14 (-99.5749, -85.7498) -> (-97.0749, -85.7498) centre (-98.3249, -85.7498) ccw
  line L15 (-99.5749, -85.7498) -> (-99.5749, -18.2498)
  arc A15 (-97.0749, -18.2498) -> (-99.5749, -18.2498) centre (-98.3249, -18.2498) ccw
  line L16 (-117.0749, -18.2498) -> (-117.0749, -85.7498)
  arc A16 (-119.5749, -85.7498) -> (-117.0749, -85.7498) centre (-118.3249, -85.7498) ccw
  line L17 (-119.5749, -85.7498) -> (-119.5749, -18.2498)
  arc A17 (-117.0749, -18.2498) -> (-119.5749, -18.2498) centre (-118.3249, -18.2498) ccw
  circle A18 centre (-36.3235, -43.5484) radius 15
  line L18 (-19.1125, -85.625) -> (-11.1125, -85.625)
  line L19 (-11.1125, -85.625) -> (-11.1125, -99.625)
  arc A19 (-19.1125, -99.625) -> (-11.1125, -99.625) centre (-15.1125, -99.625) ccw
  line L20 (-19.1125, -99.625) -> (-19.1125, -85.625)
  circle A20 centre (-119.8875, -99.625) radius 4
  line L21 (3.0749, 6.5583) -> (-128.0749, 6.5583)
  arc A21 (-132.0749, 2.5583) -> (-128.0749, 6.5583) centre (-128.0749, 2.5583) ccw
  line L22 (-132.0749, 2.5583) -> (-132.0749, -106.5583)
  arc A22 (-128.0749, -110.5583) -> (-132.0749, -106.5583) centre (-128.0749, -106.5583) ccw
  line L23 (-128.0749, -110.5583) -> (3.0749, -110.5583)
  arc A23 (7.0749, -106.5583) -> (3.0749, -110.5583) centre (3.0749, -106.5583) ccw
  line L24 (7.0749, -106.5583) -> (7.0749, 2.5583)
  arc A24 (3.0749, 6.5583) -> (7.0749, 2.5583) centre (3.0749, 2.5583) ccw
  circle A25 centre (-15.1125, -4.375) radius 4
  circle A26 centre (-119.8875, -4.375) radius 4
  line L25 (-117.3025, -102.6775) -> (-125.4899, -109.6108)
  line L26 (-122.4725, -96.5725) -> (-130.6599, -103.5058)
  arc A27 (-125.4899, -109.6108) -> (-130.6599, -103.5058) centre (-128.0749, -106.5583) ccw
  arc A28 (-122.4725, -96.5725) -> (-117.3025, -102.6775) centre (-119.8875, -99.625) ccw
  line L27 (-122.4725, -7.4275) -> (-130.6599, -0.4942)
  line L28 (-117.3025, -1.3225) -> (-125.4899, 5.6108)
  arc A29 (-117.3025, -1.3225) -> (-122.4725, -7.4275) centre (-119.8875, -4.375) ccw
  arc A30 (-130.6599, -0.4942) -> (-125.4899, 5.6108) centre (-128.0749, 2.5583) ccw
  circle A31 centre (-15.1125, -4.375) radius 5.25
  dimension "d295" = 10.5
  constraint coincident A20 L25.start
  constraint coincident A22 L25.end
  constraint tangent A22 L25
  constraint tangent A20 L25
  constraint coincident A20 L26.start
  constraint coincident A22 L26.end
  constraint tangent A22 L26
  constraint tangent A20 L26
  constraint tangent L26 A28
  constraint coincident A26 L27.start
  constraint coincident A21 L27.end
  constraint tangent A21 L27
  constraint coincident A26 L28.start
  constraint coincident A21 L28.end
  constraint tangent A21 L28
  constraint tangent A26 L28
  constraint tangent A26 L27
  constraint tangent L28 A29
  constraint concentric A25 A31
  measures "d295" diameter of A31
extrude "Extrude12" add sketch "STRENGHTEN" along normal up to surface (47.5 mm away) contours A20 A22 L25 L26 A27 A28 | A21 A26 L27 L28 A29 A30
extrude "Extrude13" add sketch "STRENGHTEN" along normal blind 4.5 contours A31
fillet "Fillet2" radius 4.5 1 edges at (20.0072, 6.2735, 6.5)
extrude "Extrude8" [rolled back] side1offset 0 taper angle 0
equation "d28 = ( ( 104.775 / 2 ) * 1 mm ) - 5 * 1 mm"
equation "d29 = ( 95.25 / 2 ) * 1 mm"
equation "d195 = ( 117.117 / 2 ) * 1 mm"

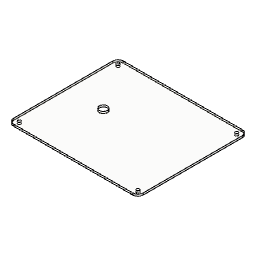
design "Cover"
Autodesk Fusion 360 part; units mm, degrees
sketch "Sketch1" plane through (0, 0, 0) normal (0, 0, 1) x (1, 0, 0)
  line L0 (62.5, 54.9936) -> (62.5, 47.4797) construction
  line L1 (125, 0) -> (125, 104)
  line L2 (0, 104) -> (125, 0) construction
  line L3 (-7.0749, -2.5583) -> (-7.0749, 106.5583)
  line L4 (0, 104) -> (0, 0)
  line L5 (134.0749, -2.8083) -> (134.0749, 106.8083)
  circle A0 centre (-3.0749, 106.5583) radius 1.75
  line L6 (60.7161, 52) -> (65.2538, 52) construction
  line L7 (-9.0749, -2.8083) -> (-9.0749, 106.8083)
  line L8 (-3.0749, 110.5583) -> (128.0749, 110.5583)
  line L9 (125, 104) -> (0, 104)
  arc A1 (134.0749, 106.8083) -> (128.3249, 112.5583) centre (128.3249, 106.8083) ccw
  line L10 (132.0749, -2.5583) -> (132.0749, 106.5583)
  line L11 (12.9183, 93.252) -> (-22.6564, 122.8501) construction
  line L12 (12.9183, 10.748) -> (-22.6564, -18.8501) construction
  line L13 (125, 104) -> (0, 0) construction
  arc A2 (-3.0749, -6.5583) -> (-7.0749, -2.5583) centre (-3.0749, -2.5583) ccw
  line L14 (112.0817, 10.748) -> (147.6564, -18.8501) construction
  circle A3 centre (128.0749, -2.5583) radius 1.75
  line L15 (112.0817, 93.252) -> (147.6564, 122.8501) construction
  line L16 (-7.0749, -2.5583) -> (-7.0749, -7.9197) construction
  arc A4 (-7.0749, 106.5583) -> (-3.0749, 110.5583) centre (-3.0749, 106.5583) ccw
  arc A5 (128.0749, 110.5583) -> (132.0749, 106.5583) centre (128.0749, 106.5583) ccw
  line L17 (-3.3249, 112.5583) -> (128.3249, 112.5583)
  circle A6 centre (128.0749, 106.5583) radius 1.75
  line L18 (-3.3249, -8.5583) -> (128.3249, -8.5583)
  arc A7 (132.0749, -2.5583) -> (128.0749, -6.5583) centre (128.0749, -2.5583) ccw
  arc A8 (-9.0749, -2.8083) -> (-3.3249, -8.5583) centre (-3.3249, -2.8083) ccw
  line L19 (0, 0) -> (125, 0)
  line L20 (-3.0749, -6.5583) -> (128.0749, -6.5583)
  line L21 (132.0749, -2.5583) -> (132.0749, -5.8863) construction
  circle A9 centre (-3.0749, -2.5583) radius 1.75
  arc A10 (-3.3249, 112.5583) -> (-9.0749, 106.8083) centre (-3.3249, 106.8083) ccw
  arc A11 (128.3249, -8.5583) -> (134.0749, -2.8083) centre (128.3249, -2.8083) ccw
  dimension "d1" = 125
  dimension "d2" = 104
  dimension "d3" = 8
  dimension "d4" = 3.5
  dimension "d6" = 5.75
  dimension "d7" = 5.75
  dimension "d8" = 5.75
  dimension "d9" = 5.75
  constraint horizontal L19
  constraint vertical L1
  constraint horizontal L9
  constraint vertical L4
  constraint coincident L4.end L13.end
  constraint coincident L15.start L13
  constraint parallel L13 L15
  constraint coincident A5.centre L15
  constraint concentric A5 A6
  constraint coincident L1.end A5
  constraint vertical L0
  constraint perpendicular L0 L6
  constraint symmetric L15.start L11.start L0
  constraint symmetric L15.end L11.end L0
  constraint symmetric L0 A4 A5
  constraint symmetric L0 A0 A6
  constraint symmetric L15.start L14.start L6
  constraint symmetric L15.end L14.end L6
  constraint symmetric L6 A5 A7
  constraint symmetric L6 A3 A6
  constraint symmetric L6 A2 A4
  constraint symmetric L12.start L11.start L6
  constraint symmetric L12.end L11.end L6
  constraint symmetric A0 L6 A9
  constraint horizontal L8
  constraint tangent L8 A5
  constraint horizontal L20
  constraint tangent A7 L20
  constraint coincident L4.end A2
  constraint tangent A2 L16
  constraint perpendicular L16 L20
  constraint perpendicular L3 L8
  constraint tangent A7 L21
  constraint perpendicular L20 L21
  constraint parallel L8 L17
  constraint parallel L3 L7
  constraint parallel L18 L20
  constraint coincident L21.end L14
  constraint tangent L17 A10
  constraint tangent L7 A10
  constraint tangent L7 A8
  constraint tangent L18 A8
  constraint tangent L5 A11
  constraint tangent L18 A11
  constraint tangent A1 L17
  constraint tangent L5 A1
  measures "d1" distance of L1.start L4.end
  measures "d2" distance of L2.start L4.end
  measures "d3" diameter of A5
  measures "d4" diameter of A6
  measures "d6" radius of A10
  measures "d7" radius of A8
  measures "d8" radius of A11
  measures "d9" radius of A1
extrude "Extrude1" add sketch "Sketch1" along normal blind 2 contours L1 L4 L9 L19 | L1 L10 A5 A7 | A2 A7 L19 L20 | L8 L9 A4 A5 | L3 L4 A2 A4 | L5 L7 A1 L17 L18 A8 A10 A11
sketch "Sketch2" plane through (0, 0, 2) normal (0, 0, 1) x (-1, 0, 0)
  circle A0 centre (3.0749, 2.5583) radius 1.75
  circle A1 centre (3.0749, -106.5583) radius 1.75
  circle A2 centre (-128.0749, -106.5583) radius 1.75
  circle A3 centre (-128.0749, 2.5583) radius 1.75
  arc A4 (9.0749, 2.8083) -> (3.3249, 8.5583) centre (3.3249, 2.8083) ccw
  line L0 (3.3249, 8.5583) -> (-128.3249, 8.5583)
  arc A5 (-128.3249, 8.5583) -> (-134.0749, 2.8083) centre (-128.3249, 2.8083) ccw
  line L1 (-134.0749, 2.8083) -> (-134.0749, -106.8083)
  arc A6 (-134.0749, -106.8083) -> (-128.3249, -112.5583) centre (-128.3249, -106.8083) ccw
  line L2 (-128.3249, -112.5583) -> (3.3249, -112.5583)
  arc A7 (3.3249, -112.5583) -> (9.0749, -106.8083) centre (3.3249, -106.8083) ccw
  line L3 (9.0749, -106.8083) -> (9.0749, 2.8083)
  circle A8 centre (-30.9209, -56.3953) radius 4.5
  dimension "d12" = 9
  dimension "d13" = 56.163
  dimension "d14" = 103.154
  measures "d12" diameter of A8
  measures "d13" distance of L2 A8.centre
  measures "d14" distance of L1 A8.centre
extrude "Extrude2" cut sketch "Sketch2" against normal up to surface (2 mm away) contours A8
equation "d13 = 52.663 mm + 3.5 mm"
equation "d14 = 99.654 mm + 3.5 mm"
